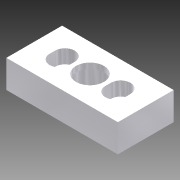
# Autodesk Inventor part: 13_0204_057
Saved by Autodesk Inventor 2012 SP1 (Build 160190100, 190)
## iProperties
Created: 2013-04-15
Part Number: 13_0204_057
Material: Default
Document SubType Name: Modeling
Designer: vogel
Density: 1 g/cm^3
Author: vogel
Autodesk Inventor part; units mm, degrees
ref_plane "YZ Plane" through (0, 0, 0) normal (1, 0, 0) x (0, 1, 0)
ref_plane "XZ Plane" through (0, 0, 0) normal (0, 1, 0) x (-1, 0, 0)
ref_plane "XY Plane" through (0, 0, 0) normal (0, 0, 1) x (1, 0, 0)
sketch "Skizze1" plane through (0, 0, 0) normal (0, 0, 1) x (1, 0, 0)
  line L0 (-20, 10) -> (20, 10)
  line L1 (20, 10) -> (20, -10)
  line L2 (20, -10) -> (-20, -10)
  line L3 (-20, -10) -> (-20, 10)
  line L4 (-28, 0) -> (28, 0) projected
  line L5 (0, -14) -> (0, 14) projected
  circle A0 centre (0, 0) radius 5
  dimension "d0" = 40
  dimension "d1" = 20
  dimension "d2" = 10
  constraints: 8 end point, 2 parallel, 1 centre point, 1 coincident, 1 horizontal, 1 perpendicular, 2 other
  measures "d0" distance of L0.start L0.end
  measures "d1" distance of L2.end L0.start
  measures "d2" diameter of A0
extrude "Extrusion1" add sketch "Skizze1" along normal blind 10 contours L0 L5 A0 L4 L3 | L0 L1 L4 A0 L5 | L4 A0 L5 L2 L3 | L1 L2 L5 A0 L4
sketch "Skizze2" plane through (0, 0, 0) normal (0, 0, -1) x (-1, 0, 0)
  circle A0 centre (0, 0) radius 5 projected
  circle A1 centre (0, 0) radius 6
  dimension "d5" = 12
  constraints: 1 centre point, 1 coincident
  measures "d5" diameter of A1
extrude "Extrusion2" cut sketch "Skizze2" against normal blind 8
sketch "Skizze3" plane through (0, 0, 10) normal (0, 0, 1) x (1, 0, 0)
  line L0 (-20, 10) -> (20, 10) projected
  line L1 (20, -10) -> (-20, -10) projected
  line L2 (-13, 10) -> (-13, -10)
  line L3 (13, -10) -> (13, 10)
  line L4 (-11.2, 1) -> (-11.2, -1)
  line L5 (-14.8, -1) -> (-14.8, 1)
  line L6 (14.8, 1) -> (14.8, -1)
  line L7 (11.2, -1) -> (11.2, 1)
  line L8 (-28, 0) -> (28, 0) projected
  line L9 (0, -14) -> (0, 14) projected
  arc A0 (-11.2, 1) -> (-14.8, 1) centre (-13, 1) ccw
  arc A1 (-14.8, -1) -> (-11.2, -1) centre (-13, -1) ccw
  arc A2 (11.2, -1) -> (14.8, -1) centre (13, -1) ccw
  arc A3 (14.8, 1) -> (11.2, 1) centre (13, 1) ccw
  dimension "d8" = 26
  dimension "d9" = 3.6
  dimension "d11" = 2
  constraints: 12 end point, 8 point on circle, 8 tangent, 4 centre point, 4 parallel, 4 point on line, 2 symmetric about line, 1 equal radius, 1 perpendicular, 3 other
  measures "d8" distance between parallel lines of L3 L2
  measures "d9" distance between parallel lines of L5 L4
  measures "d11" distance of A1.centre A0.centre
extrude "Extrusion3" cut sketch "Skizze3" against normal through all contours A0 L4 L8 L2 | L2 L8 L5 A0 | L8 L4 A1 L2 | L2 A1 L5 L8 | A3 L6 L8 L3 | L3 L8 L7 A3 | L8 L3 A2 L7 | L8 L6 A2 L3
sketch "Skizze4" plane through (0, 0, 10) normal (0, 0, 1) x (1, 0, 0)
  arc A0 (-14.8, -1) -> (-11.2, -1) centre (-13, -1) ccw projected
  line L0 (-14.8, -1) -> (-14.8, 1) projected
  arc A1 (-11.2, 1) -> (-14.8, 1) centre (-13, 1) ccw projected
  line L1 (-11.2, 1) -> (-11.2, -1) projected
  arc A2 (11.2, -1) -> (14.8, -1) centre (13, -1) ccw projected
  line L2 (11.2, -1) -> (11.2, 1) projected
  arc A3 (14.8, 1) -> (11.2, 1) centre (13, 1) ccw projected
  line L3 (14.8, 1) -> (14.8, -1) projected
  line L4 (-16.5, 1) -> (-16.5, -1)
  arc A4 (-16.5, -1) -> (-9.5, -1) centre (-13, -1) ccw
  line L5 (-9.5, -1) -> (-9.5, 1)
  arc A5 (-9.5, 1) -> (-16.5, 1) centre (-13, 1) ccw
  line L6 (9.5, 1) -> (9.5, -1)
  arc A6 (9.5, -1) -> (16.5, -1) centre (13, -1) ccw
  line L7 (16.5, -1) -> (16.5, 1)
  arc A7 (16.5, 1) -> (9.5, 1) centre (13, 1) ccw
  dimension "d14" = 7
  constraints: 8 end point, 8 point on circle, 4 centre point, 1 equal radius, 6 other
  measures "d14" distance between parallel lines of L7 L6
extrude "Extrusion4" cut sketch "Skizze4" against normal blind 5
